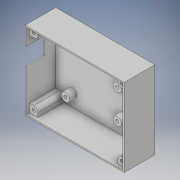
# Autodesk Inventor part: case_bottom
Saved by Autodesk Inventor 2019 (Build 230136000, 136)
## iProperties
Created: 2019-03-24
Part Number: case_bottom
Material: Generic
Document SubType Name: Modeling
Designer: janza
Density: 1 g/cm^3
Appearance: Default
Author: janza
Autodesk Inventor part; units mm, degrees
ref_plane "YZ Plane" through (0, 0, 0) normal (1, 0, 0) x (0, 1, 0)
ref_plane "XZ Plane" through (0, 0, 0) normal (0, 1, 0) x (-1, 0, 0)
sketch "Zakladna" plane through (0, 0, 0) normal (0, 0, 1) x (1, 0, 0)
  line L0 (0, 0) -> (92, 0)
  line L1 (92, 0) -> (92, 72)
  line L2 (92, 72) -> (0, 72)
  line L3 (0, 72) -> (0, 0)
  dimension "d0" = 92
  dimension "d1" = 72
  constraints: 8 end point, 2 parallel, 1 horizontal, 1 perpendicular
  measures "d0" distance of L2.end L1.end
  measures "d1" distance of L1.end L0.end
extrude "Extrusion1" add sketch "Zakladna" along normal blind 1.2
sketch "Steny" plane through (0, 0, 1.2) normal (0, 0, 1) x (1, 0, 0)
  line L0 (0, 0) -> (92, 0) projected
  line L1 (0, 8) -> (0, 0)
  line L2 (0, 0) -> (8, 0)
  line L3 (0, 0) -> (8, 0)
  line L4 (0, 72) -> (8, 72)
  line L5 (0, 72) -> (8, 72)
  line L6 (92, 0) -> (92, 72) projected
  line L7 (0, 56.55) -> (-1.2, 56.55)
  line L8 (-1.2, 39.75) -> (-1.2, 0)
  line L9 (-1.2, 0) -> (-1.2, -1.2)
  line L10 (-1.2, -1.2) -> (0, -1.2)
  line L11 (0, 0) -> (0, 39.75)
  line L12 (92, 72) -> (0, 72) projected
  line L13 (0, 73.2) -> (-1.2, 73.2)
  line L14 (-1.2, 73.2) -> (-1.2, 56.55)
  line L15 (0, 72) -> (92, 72)
  line L16 (93.2, 72) -> (93.2, 73.2)
  line L17 (93.2, 73.2) -> (0, 73.2)
  line L18 (92, 72) -> (92, 0)
  line L19 (92, -1.2) -> (93.2, -1.2)
  line L20 (93.2, -1.2) -> (93.2, 72)
  line L21 (92, -1.2) -> (0, -1.2)
  line L22 (-1.2, 39.75) -> (0, 39.75)
  line L23 (0, 56.55) -> (0, 72)
  point P0 (8, 4)
  dimension "d15" = 1.2
  dimension "d16" = 16.8
  dimension "d17" = 1.2
  dimension "d18" = 1.2
  dimension "d19" = 1.2
  dimension "d20" = 1.2
  dimension "d21" = 1.2
  dimension "d23" = 1.2
  constraints: 42 end point, 6 point on line, 4 perpendicular, 3 vertical, 2 collinear, 2 horizontal
  measures "d15" distance of L7.start L7.end
  measures "d16" distance of L7.end L8.start
  measures "d17" distance of L8.end L9.end
  measures "d18" distance of L4.start L13.start
  measures "d19" distance of L13.start L13.end
  measures "d20" distance of L6.end L16.start
  measures "d21" distance of L16.start L16.end
  measures "d23" distance of L19.start L19.end
sketch "Uchyt_arduino" plane through (0, 0, 1.2) normal (0, 0, 1) x (1, 0, 0)
  circle A0 centre (16.2, 12) radius 4
  circle A1 centre (16.2, 12) radius 1.5
  circle A2 centre (16.2, 60) radius 4
  circle A3 centre (16.2, 60) radius 1.5
  circle A4 centre (65.5, 44.75) radius 4
  circle A5 centre (65.5, 44.75) radius 1.5
  circle A6 centre (65.5, 16.75) radius 4
  circle A7 centre (65.5, 16.75) radius 1.5
  circle A8 centre (16.2, 12) radius 4
  circle A9 centre (16.2, 12) radius 1.5
  circle A10 centre (16.2, 60) radius 4
  circle A11 centre (16.2, 60) radius 1.5
  circle A12 centre (65.5, 44.75) radius 4
  circle A13 centre (65.5, 44.75) radius 1.5
  circle A14 centre (65.5, 16.75) radius 4
  circle A15 centre (65.5, 16.75) radius 1.5
  point P0 (0, 0)
  dimension "d31" = 8
  dimension "d32" = 3
  dimension "d33" = 8
  dimension "d34" = 3
  dimension "d35" = 8
  dimension "d36" = 3
  dimension "d37" = 8
  dimension "d38" = 3
  dimension "d39" = 8
  dimension "d40" = 3
  dimension "d41" = 8
  dimension "d42" = 3
  constraints: 16 centre point, 8 coincident
  measures "d31" diameter of A0
  measures "d32" diameter of A1
  measures "d33" diameter of A4
  measures "d34" diameter of A5
  measures "d35" diameter of A6
  measures "d36" diameter of A7
  measures "d37" diameter of A8
  measures "d38" diameter of A9
  measures "d39" diameter of A12
  measures "d40" diameter of A13
  measures "d41" diameter of A14
  measures "d42" diameter of A15
sketch "Stena_RJ45" plane through (0, 0, 1.2) normal (0, 0, 1) x (1, 0, 0)
  line L0 (0, 56.55) -> (-1.2, 56.55) projected
  line L1 (-1.2, 39.75) -> (0, 39.75) projected
  line L2 (0, 36) -> (0, 62.75) projected
  line L3 (-1.2, 56.55) -> (-1.2, 39.75)
  line L4 (0, 39.75) -> (-1.2, 39.75)
  line L5 (0, 39.75) -> (0, 56.55)
  line L6 (0, 72) -> (0, 0) projected
  constraints: 6 end point, 2 collinear, 1 perpendicular
sketch "Spojeni_srouby" plane through (0, 0, 1.2) normal (0, 0, 1) x (1, 0, 0)
  line L0 (8, 4) -> (8, 0) projected
  arc A0 (8, 4) -> (4, 8) centre (4, 4) ccw projected
  line L1 (4, 8) -> (0, 8) projected
  circle A1 centre (4, 4) radius 1.5 projected
  line L2 (0, 72) -> (0, 0) projected
  line L3 (0, 8) -> (0, 0)
  line L4 (0, 0) -> (8, 0)
  line L5 (0, 0) -> (92, 0)
  line L6 (92, 0) -> (92, 36)
  line L7 (92, 0) -> (92, 72)
  line L8 (8, 68) -> (8, 72)
  arc A2 (4, 64) -> (8, 68) centre (4, 68) ccw
  line L9 (4, 64) -> (0, 64)
  circle A3 centre (4, 68) radius 1.5
  line L10 (0, 0) -> (0, 72)
  line L11 (0, 64) -> (0, 72)
  line L12 (0, 72) -> (8, 72)
  line L13 (0, 72) -> (92, 72)
  line L14 (84, 4) -> (84, 0)
  arc A4 (88, 8) -> (84, 4) centre (88, 4) ccw
  line L15 (88, 8) -> (92, 8)
  circle A5 centre (88, 4) radius 1.5
  line L16 (92, 72) -> (92, 0)
  line L17 (92, 8) -> (92, 0)
  line L18 (92, 0) -> (84, 0)
  line L19 (92, 0) -> (0, 0)
  line L20 (84, 68) -> (84, 72)
  arc A6 (84, 68) -> (88, 64) centre (88, 68) ccw
  line L21 (88, 64) -> (92, 64)
  circle A7 centre (88, 68) radius 1.5
  line L22 (92, 0) -> (92, 72)
  line L23 (92, 64) -> (92, 72)
  line L24 (92, 72) -> (84, 72)
  line L25 (92, 72) -> (0, 72)
  constraints: 46 end point, 6 centre point, 6 point on circle, 1 midpoint, 1 perpendicular, 1 vertical
extrude "Extrusion2" add sketch "Uchyt_arduino" along normal blind 7
extrude "Extrusion3" add sketch "Steny" along normal blind 28 and the other way blind 1.2
extrude "Extrusion4" add sketch "Stena_RJ45" along normal blind 10.9 and the other way blind 1.2
extrude "Extrusion5" add sketch "Spojeni_srouby" along normal blind 25 contours L0 L4 L2 L1 A0 | L14 A4 L15 L6 L5 | L2 L12 L8 A2 L9 | L21 A6 L20 L13 L7
sketch "Sketch6" plane through (4, 4, 1.2) normal (0, 0, 1) x (1, 0, 0)
  circle A0 centre (0, 64) radius 1.5 projected
  point P0 (-4, -4)
  point P1 (0.3313, 0.2345)
  point P2 (84.6618, 64.0382)
  point P3 (84.4144, -0.0051)
  constraints: 1 coincident
hole "Hole1" at (4, 68, 1.2) at (4.3313, 4.2345, 1.2) at (88.6618, 68.0382, 1.2) at (88.4144, 3.9949, 1.2) direction (0, 0, -1) diameter 3 end through all
sketch "napajeni_znacka1" plane through (-1.2, -1.2, 0) normal (-1, 0, 0) x (0, 0, 1)
  line L0 (12.1, 57.75) -> (12.1, 40.95) projected
  line L1 (0, 0) -> (29.2, 0) projected
  circle A0 centre (20.1, 32.95) radius 0.35
  point P0 (0, 1.2)
  dimension "d65" = 0.7
  constraints: 1 centre point
  measures "d65" diameter of A0
ref_plane "napajeni_znacka2_rovina" through (-0.7, -1.2, 0) normal (-1, 0, 0) x (0, 0, 1)
sketch "napajeni_znacka2" plane through (-0.7, -1.2, 0) normal (-1, 0, 0) x (0, 0, 1)
  point P0 (0, 1.2)
  point P1 (20.1, 32.95)
  point P2 (20.1, 32.95)
  constraints: 1 coincident
loft "Loft1" cut profiles "napajeni_znacka1" section 2 point at (-0.7, 31.75, 20.1)
body "Solid1"
